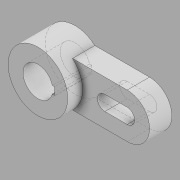
# Autodesk Inventor part: Lab2A01209499P19
Saved by Autodesk Inventor 2020 (Build 240168000, 168)
## iProperties
Created: 2019-08-22
Part Number: Lab2A01209499P19
Material: Genérico
Document SubType Name: Modeling
Designer: gerar
Density: 1 g/cm^3
Appearance: Valor por defecto
Author: gerar
Autodesk Inventor part; units mm, degrees
ref_plane "YZ Plane" through (0, 0, 0) normal (1, 0, 0) x (0, 1, 0)
ref_plane "XZ Plane" through (0, 0, 0) normal (0, 1, 0) x (-1, 0, 0)
ref_plane "XY Plane" through (0, 0, 0) normal (0, 0, 1) x (1, 0, 0)
sketch "Boceto1" plane through (0, 0, 0) normal (0, 0, 1) x (1, 0, 0)
  circle A0 centre (0, 0) radius 40
  arc A1 (19.3649, 5) -> (19.3649, -5) centre (0, 0) ccw
  line L0 (19.3649, -5) -> (22.5, -5)
  line L1 (22.5, -5) -> (22.5, 5)
  line L2 (22.5, 5) -> (19.3649, 5)
  line L3 (17.5, 0) -> (22.5, 5) construction
  line L4 (22.5, -5) -> (17.5, 0) construction
  line L5 (0, 0) -> (181.7568, 0) construction
  line L6 (26.4575, -30) -> (100, -30)
  line L7 (130, 0) -> (130, 0)
  line L8 (100, 30) -> (26.4575, 30)
  line L9 (0, -30) -> (130, 30) construction
  line L10 (130, -30) -> (0, 30) construction
  arc A2 (130, 0) -> (100, 30) centre (100, 0) ccw
  arc A3 (100, -30) -> (130, 0) centre (100, 0) ccw
  line L11 (70, -10) -> (100, -10)
  line L12 (110, 0) -> (110, 0)
  line L13 (100, 10) -> (70, 10)
  line L14 (60, 0) -> (60, 0)
  line L15 (60, -10) -> (110, 10) construction
  line L16 (110, -10) -> (60, 10) construction
  arc A4 (110, 0) -> (100, 10) centre (100, 0) ccw
  arc A5 (100, -10) -> (110, 0) centre (100, 0) ccw
  arc A6 (60, 0) -> (70, -10) centre (70, 0) ccw
  arc A7 (70, 10) -> (60, 0) centre (70, 0) ccw
  point P0 (65, 0)
  point P1 (85, 0)
  point P2 (60, 0)
  dimension "d0" = 80
  dimension "d1" = 40
  dimension "d3" = 10
  dimension "d4" = 130
  dimension "d5" = 60
  dimension "d7" = 30
  dimension "d8" = 50
  dimension "d9" = 20
  dimension "d10" = 85
  dimension "d11" = 10
  dimension "d12" = 10
  constraints: 34 end point, 16 point on circle, 14 point on line, 12 tangent, 8 centre point, 5 parallel, 4 horizontal, 4 midpoint, 3 equal radius, 3 perpendicular, 2 coincident
  measures "d0" diameter of A0
  measures "d1" diameter of A1
  measures "d3" distance of L1.end L0.end
  measures "d4" distance of L10.end L9.end
  measures "d5" distance of L9.end L10.start
  measures "d7" radius of A2
  measures "d8" distance of L16.end L15.end
  measures "d9" distance of L15.end L16.start
  measures "d10" distance of point (85, 0) L5.start
  measures "d11" radius of A4
  measures "d12" radius of A7
extrude "Extrusión1" add sketch "Boceto1" along normal blind 30
sketch "Boceto2" plane through (0, 0, 30) normal (0, 0, 1) x (1, 0, 0)
  arc A0 (26.4575, 30) -> (26.4575, -30) centre (0, 0) ccw projected
  circle A1 centre (0, 0) radius 40
  arc A2 (19.3649, 5) -> (20, 0) centre (0, 0) ccw
  line L0 (19.3649, 5) -> (22.5, 5)
  line L1 (22.5, 5) -> (22.5, -5)
  line L2 (22.5, -5) -> (19.3649, -5)
  line L3 (18.5, 3) -> (22.5, -5) construction
  line L4 (22.5, 5) -> (20.3695, 0.739) construction
  point P0 (26.4575, -30)
  dimension "d16" = 10
  dimension "d18" = 0
  constraints: 10 end point, 3 point on circle, 2 coincident, 2 point on line, 1 centre point, 1 horizontal, 1 parallel, 1 perpendicular, 3 other
  measures "d16" distance of L0.end L1.end
  measures "d18" vertical distance of point (0, 0) A2.end
extrude "Extrusión2" add sketch "Boceto2" along normal blind 20
